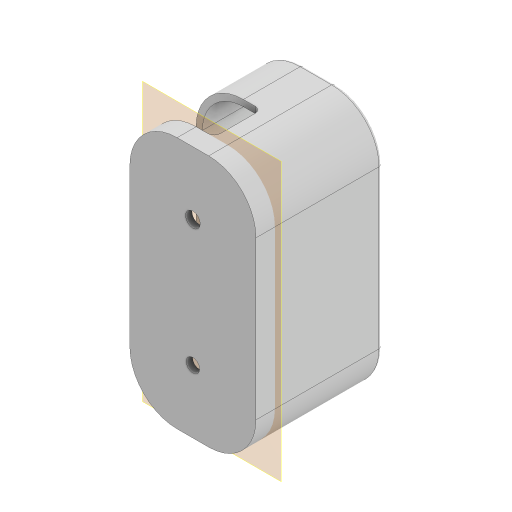
# Autodesk Inventor part: lock-case
Saved by Autodesk Inventor 2024 (Build 280153000, 153)
## iProperties
Created: 2023-09-16
Part Number: lock-case
Material: Generic
Document SubType Name: Modeling
Designer: draev
Density: 1 g/cm^3
Appearance: Default
Author: draev
Autodesk Inventor part; units mm, degrees
ref_plane "YZ Plane" through (0, 0, 0) normal (1, 0, 0) x (0, 1, 0)
ref_plane "XZ Plane" through (0, 0, 0) normal (0, 1, 0) x (-1, 0, 0)
ref_plane "XY Plane" through (0, 0, 0) normal (0, 0, 1) x (1, 0, 0)
sketch "Sketch1" plane through (0, 0, 0) normal (0, 0, 1) x (1, 0, 0)
  line L0 (-20.7162, 13.5128) -> (19.2838, 13.5128)
  line L1 (19.2838, 13.5128) -> (19.2838, -66.4872)
  line L2 (19.2838, -66.4872) -> (-20.7162, -66.4872)
  line L3 (-20.7162, -66.4872) -> (-20.7162, 13.5128)
  point P0 (0, 0)
  dimension "d0" = 40
  dimension "d1" = 80
  constraints: 8 end point, 2 parallel, 1 horizontal, 1 perpendicular
  measures "d0" distance of L1.end L2.end
  measures "d1" distance of L0.end L1.end
extrude "Extrusion1" add sketch "Sketch1" along normal blind 40
fillet "Fillet1" radius 15 4 edges at (-20.7162, 13.5128, 20) (19.2838, 13.5128, 20) (-20.7162, -66.4872, 20) (19.2838, -66.4872, 20)
shell "Shell1" thickness 2 removed faces 0
ref_plane "Work Plane1" through (0, 0, 34) normal (0, 0, 1) x (1, 0, 0)
sketch "Sketch3" plane through (0, 0, 34) normal (0, 0, 1) x (1, 0, 0)
  arc A0 (-5.7162, 13.5128) -> (-20.7162, -1.4872) centre (-5.7162, -1.4872) ccw projected
  line L0 (-20.7162, -1.4872) -> (-20.7162, -51.4872) projected
  line L1 (-20.7162, -51.4872) -> (0, -51.4872)
  line L2 (0, -51.4872) -> (0, 13.5128)
  line L3 (0, 13.5128) -> (-5.7162, 13.5128)
  point P0 (0, 0)
  constraints: 6 end point, 2 perpendicular, 1 horizontal, 1 tangent
extrude "Extrusion2" cut sketch "Sketch3" against normal blind 15
fillet "Fillet3" radius 2 4 edges at (0, 12.5128, 19) (0, 12.5128, 34) (-19.7162, -51.4872, 34) (-19.7162, -51.4872, 19)
sketch "Sketch4" plane through (0, 0, 40) normal (0, 0, 1) x (1, 0, 0)
  circle A0 centre (-0.7162, -46.4872) radius 2.1395
  circle A1 centre (-0.7162, -6.4872) radius 2.337
  line L0 (-20.7162, -1.4872) -> (-20.7162, -51.4872) projected
  line L1 (4.2838, 13.5128) -> (-5.7162, 13.5128) projected
  line L2 (-5.7162, -66.4872) -> (4.2838, -66.4872) projected
  point P0 (0, 0)
  dimension "d11" = 20
  dimension "d12" = 20
  dimension "d13" = 20
  dimension "d14" = 20
  constraints: 2 centre point
  measures "d11" distance from line of L0 A0.centre
  measures "d12" distance from line of L0 A1.centre
  measures "d13" distance from line of L1 A1.centre
  measures "d14" distance from line of L2 A0.centre
extrude "Extrusion3" cut sketch "Sketch4" against normal up to next
fillet "Fillet4" radius 1 8 edges at (-0.7162, 13.5128, 0) (-16.3228, 9.1194, 0) (-20.7162, -26.4872, 0) (-16.3228, -62.0938, 0) (-0.7162, -66.4872, 0) (14.8904, -62.0938, 0) (19.2838, -26.4872, 0) (14.8904, 9.1194, 0)
body "Solid1"
